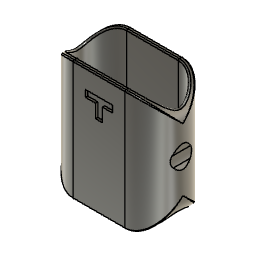
airpods (Autodesk Fusion 360 design; units mm, degrees)
Autodesk Fusion 360 part; units mm, degrees
note: some values were not read from the file. Set by a fixed rule: which sketch regions a step uses.
sketch "Sketch1" plane through (0, 0, 0) normal (0, 0, 1) x (1, 0, 0)
  line L0 (0, 0) -> (48.8, 0)
  line L1 (48.8, 0) -> (48.8, 25.8)
  line L2 (48.8, 25.8) -> (0, 25.8)
  line L3 (0, 25.8) -> (0, 0)
  dimension "d1" = 48.8
  dimension "d2" = 25.8
  constraint horizontal L0
  constraint vertical L1
  constraint horizontal L2
  constraint vertical L3
  constraint coincident L0.start L3.end
  measures "d1" distance of L0.start L0.end
  measures "d2" distance of L0.start L2.end
extrude "Extrude1" add sketch "Sketch1" along normal blind 53.5
fillet "Fillet1" radius 12.9 2 faces at (48.8, 8.6, 35.6667) (0, 17.2, 35.6667)
sketch "Sketch6" plane through (0, 0, 53.5) normal (0, 0, 1) x (-1, 0, 0)
  line L0 (-12.9, -25.8) -> (-12.9, 0)
  line L1 (-12.9, 0) -> (-35.9, 0)
  line L2 (-35.9, 0) -> (-35.9, -25.8)
  line L3 (-35.9, -25.8) -> (-12.9, -25.8)
  line L4 (-12.9, -23.8) -> (-35.9, -23.8)
  line L5 (-46.8, -12.9) -> (-46.8, -12.9)
  line L6 (-35.9, -2) -> (-12.9, -2)
  line L7 (-2, -12.9) -> (-2, -12.9)
  line L8 (0, -15.15) -> (0, -10.65)
  arc A0 (-12.9, -23.8) -> (-2, -12.9) centre (-12.9, -12.9) ccw
  arc A1 (-2, -12.9) -> (-12.9, -2) centre (-12.9, -12.9) ccw
  arc A2 (-46.8, -12.9) -> (-35.9, -23.8) centre (-35.9, -12.9) ccw
  arc A3 (-35.9, -2) -> (-46.8, -12.9) centre (-35.9, -12.9) ccw
  point P0 (-2, -23.8)
  point P1 (-46.8, -23.8)
  point P2 (-2, -2)
  dimension "d47" = 44.8
  dimension "d48" = 21.8
  dimension "d49" = 2
  dimension "d51" = 10.9
  dimension "d52" = 10.9
  dimension "d53" = 10.9
  dimension "d54" = 10.9
  constraint horizontal L4
  constraint horizontal L6
  constraint coincident P0 L4
  constraint tangent L4 A0
  constraint coincident P2 L6
  constraint coincident P2 L7
  constraint tangent L6 A1
  constraint coincident P1 L4
  constraint tangent L4 A2
  constraint tangent L6 A3
  measures "d47" distance of P0 P1
  measures "d48" distance of P0 P2
  measures "d49" distance of L3 L4
  measures "d51" radius of A0
  measures "d52" radius of A1
  measures "d53" radius of A2
  measures "d54" radius of A3
extrude "Extrude6" cut sketch "Sketch6" against normal blind 51.5 contours L0 L2 L4 L6 | L0 A0 A1 | L2 A2 A3
sketch "Sketch3" plane through (0, 0, 0) normal (0, -1, 0) x (1, 0, 0)
  line L0 (12.9, 0) -> (35.9, 0)
  line L1 (35.9, 0) -> (35.9, 53.5)
  line L2 (35.9, 53.5) -> (12.9, 53.5)
  line L3 (24.4, 45.004) -> (30.4, 45.004)
  line L4 (24.4, 45.004) -> (18.4, 45.004)
  line L5 (18.4, 45.004) -> (18.4, 42.004)
  line L6 (18.4, 42.004) -> (22.9, 42.004)
  line L7 (22.9, 42.004) -> (22.9, 36.004)
  line L8 (22.9, 36.004) -> (25.9, 36.004)
  line L9 (25.9, 36.004) -> (25.9, 42.004)
  line L10 (25.9, 42.004) -> (30.4, 42.004)
  line L11 (30.4, 42.004) -> (30.4, 45.004)
  line L12 (12.9, 53.5) -> (12.9, 0)
  dimension "d17" = 6
  dimension "d18" = 6
  dimension "d19" = 3
  dimension "d20" = 4.5
  dimension "d21" = 6
  dimension "d22" = 3
  dimension "d23" = 4.5
  dimension "d57" = 10
  constraint parallel L3 L4
  constraint perpendicular L4 L5
  constraint perpendicular L5 L6
  constraint perpendicular L6 L7
  constraint perpendicular L7 L8
  constraint perpendicular L8 L9
  constraint perpendicular L9 L10
  measures "d17" distance of L3.start L3.end
  measures "d18" distance of L3.start L4.end
  measures "d19" distance of L4.end L5.end
  measures "d20" distance of L5.end L6.end
  measures "d21" distance of L6.end L7.end
  measures "d22" distance of L7.end L8.end
  measures "d23" distance of L9.end L10.end
  measures "d57" distance of L1 L9
extrude "Extrude7" cut sketch "Sketch3" against normal blind 1 contours L3 L4 L5 L6 L7 L8 L9 L10 L11
fillet "Fillet4" radius 0.5 4 edges at (24.4, 2, 53.5) (2, 12.9, 47.4993) (24.4, 23.8, 53.5) (46.8, 12.9, 47.4993)
fillet "Fillet5" radius 0.5 6 edges at (3.7783, 3.7783, 49.7217) (24.4, 0, 53.5) (45.0217, 3.7783, 49.7217) (45.0217, 22.0217, 49.7217) (24.4, 25.8, 53.5) (3.7783, 22.0217, 49.7217)
sketch "Sketch7" plane through (0, 0, 0) normal (0, -1, 0) x (1, 0, 0)
  line L0 (35.9, 53) -> (12.9, 53)
  line L1 (12.9, 53) -> (12.9, 0)
  line L2 (12.9, 0) -> (35.9, 0)
  line L3 (35.9, 0) -> (35.9, 53)
  line L4 (18.4, 42.004) -> (18.4, 45.004)
  line L5 (18.4, 45.004) -> (30.4, 45.004)
  line L6 (30.4, 45.004) -> (30.4, 42.004)
  line L7 (30.4, 42.004) -> (25.9, 42.004)
  line L8 (25.9, 42.004) -> (25.9, 36.004)
  line L9 (25.9, 36.004) -> (22.9, 36.004)
  line L10 (22.9, 36.004) -> (22.9, 42.004)
  line L11 (22.9, 42.004) -> (18.4, 42.004)
  line L12 (0, 28) -> (0, 33)
  line L13 (0, 28) -> (0, 23)
  line L14 (0, 23) -> (0.5681, 25.1202)
  line L15 (0.6856, 29.8094) -> (0, 33)
  arc A0 (0.5681, 25.1202) -> (0.6856, 29.8094) centre (-9.0911, 27.7084) ccw
  dimension "d64" = 5
  dimension "d65" = 5
  dimension "d66" = 15
  dimension "d67" = 10
  constraint vertical L12
  constraint parallel L12 L13
  constraint tangent L14 A0
  constraint tangent L15 A0
  measures "d64" distance of L12.start L12.end
  measures "d65" distance of L12.start L13.end
  measures "d66" angle of L13 L14
  measures "d67" radius of A0
extrude "Extrude8" cut sketch "Sketch7" against normal blind 100 contours L12 L13 L14 L15 A0
ref_plane "WorkPlane2" through (24.4, 0, 0) normal (1, 0, 0) x (0, 1, 0)
mirror "Mirror2" about plane through (24.4, 0, 0) normal (1, 0, 0) of "Extrude8"
fillet "Fillet6" radius 0.5 6 edges at (3.7783, 3.7783, 3.7783) (24.4, 0, 0) (45.0217, 3.7783, 3.7783) (45.0217, 22.0217, 3.7783) (24.4, 25.8, 0) (3.7783, 22.0217, 3.7783)
